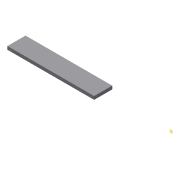
# Autodesk Inventor part: ArmBacking
Saved by Autodesk Inventor 2015 (Build 190159000, 159)
## iProperties
Created: 2015-03-07
Part Number: ArmBacking
Material: Generic
Document SubType Name: Modeling
Designer: Jaden
Density: 1 g/cm^3
Appearance: Default
Author: Jaden
Autodesk Inventor part; units mm, degrees
ref_plane "YZ Plane" through (0, 0, 0) normal (1, 0, 0) x (0, 1, 0)
ref_plane "XZ Plane" through (0, 0, 0) normal (0, 1, 0) x (-1, 0, 0)
ref_plane "XY Plane" through (0, 0, 0) normal (0, 0, 1) x (1, 0, 0)
ref_plane "Work Plane1" through (0, 0, 25.4) normal (0, 0, 1) x (1, 0, 0)
sketch "Sketch3" plane through (0, 0, 25.4) normal (0, 0, 1) x (1, 0, 0)
  line L0 (-455.2111, 54.1585) -> (-1125.1361, 54.1585)
  line L1 (-1125.1361, 54.1585) -> (-1125.1361, 79.5585)
  line L2 (-1125.1361, 79.5585) -> (-455.2111, 79.5585)
  line L3 (-455.2111, 79.5585) -> (-455.2111, 54.1585)
  circle A0 centre (-480.6111, 66.8585) radius 4.7625
  circle A1 centre (-1099.7361, 66.8585) radius 4.7625
  point P0 (0, 0)
  dimension "d8" = 669.925
  dimension "d9" = 25.4
  dimension "d11" = 9.525
  dimension "d13" = 9.525
  constraints: 8 end point, 2 centre point, 2 parallel, 1 horizontal, 1 perpendicular
  measures "d8" distance of L1.end L2.end
  measures "d9" distance of L0.end L1.end
  measures "d11" diameter of A0
  measures "d13" diameter of A1
extrude "Extrusion3" add sketch "Sketch3" along normal blind 139.7
body "Solid2"
